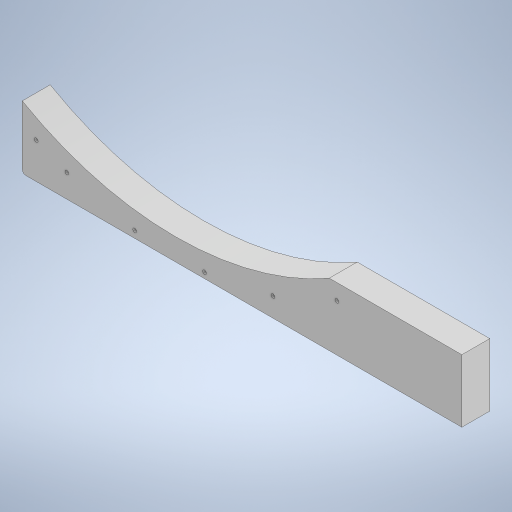
# Autodesk Inventor part: boundaryV1
Saved by Autodesk Inventor 2024.4 (Build 284460000, 460)
## iProperties
Created: 2025-11-05
Part Number: boundaryV1
Material: Generic
Document SubType Name: Modeling
Designer: jonas
Density: 1 g/cm^3
Appearance: Default
Author: jonas
Autodesk Inventor part; units mm, degrees
ref_plane "YZ Plane" through (0, 0, 0) normal (1, 0, 0) x (0, 1, 0)
ref_plane "XZ Plane" through (0, 0, 0) normal (0, 1, 0) x (-1, 0, 0)
ref_plane "XY Plane" through (0, 0, 0) normal (0, 0, 1) x (1, 0, 0)
sketch "Sketch1" plane through (0, 0, 0) normal (0, 1, 0) x (-1, 0, 0)
  line L0 (0, 329.241) -> (0, -329.241) construction
  line L1 (203.5937, 0) -> (-203.5937, 0) construction
  arc A0 (-441.1, 0) -> (220, -382.3208) centre (0, 0) ccw
  line L2 (-441.1, 0) -> (-441.1, 400)
  line L3 (-441.1, 400) -> (-500, 400)
  line L4 (-500, 400) -> (-500, -500)
  line L5 (-500, -500) -> (220, -500)
  line L6 (220, -500) -> (220, -382.3208)
  dimension "d0" = 500
  dimension "d1" = 400
  dimension "d2" = 500
  dimension "d3" = 441.1
  dimension "d4" = 720
  constraints: 14 end point, 3 perpendicular, 2 coincident, 2 midpoint, 2 point on circle, 2 vertical, 1 centre point, 1 horizontal, 1 tangent
  measures "d0" distance between parallel lines of L4 L0
  measures "d1" distance between parallel lines of L3 L1
  measures "d2" distance between parallel lines of L5 L1
  measures "d3" radius of A0
  measures "d4" distance between parallel lines of L4 L6
extrude "Extrusion1" add sketch "Sketch1" along normal blind 40
sketch "Sketch3" plane through (0, 0, 0) normal (0, -1, 0) x (1, 0, 0)
  line L0 (-480, -472.3208) -> (410, -472.3208)
  line L1 (410, -472.3208) -> (410, -382.3208)
  line L2 (410, -382.3208) -> (-480, -382.3208)
  line L3 (-480, -382.3208) -> (-480, -472.3208)
  arc A0 (-220, -382.3208) -> (441.1, 0) centre (0, 0) ccw projected
  line L4 (500, 400) -> (500, -500) projected
  line L5 (-944.7434, 629.3425) -> (927.6453, 629.3425)
  line L6 (927.6453, 629.3425) -> (927.6453, -768.0218)
  line L7 (927.6453, -768.0218) -> (-944.7434, -768.0218)
  line L8 (-944.7434, -768.0218) -> (-944.7434, 629.3425)
  dimension "d44" = 890
  dimension "d45" = 90
  dimension "d71" = 90
  constraints: 16 end point, 4 parallel, 2 horizontal, 2 perpendicular, 1 point on line
  measures "d44" distance of L1.end L2.end
  measures "d45" distance of L2.end L0.start
  measures "d71" distance between parallel lines of L4 L1
sketch "Sketch4" plane through (0, 0, 0) normal (0, -1, 0) x (1, 0, 0)
  line L0 (441.1, 400) -> (500, 400) construction
  line L1 (441.1, 0) -> (441.1, 400) construction
  arc A0 (-220, -382.3208) -> (441.1, 0) centre (0, 0) ccw construction
  line L2 (464.3817, -39.9852) -> (0, 0) construction
  line L3 (0, 0) -> (445.1648, -138.1214) construction
  line L4 (423.7332, -194.1633) -> (0, 0) construction
  line L5 (360.2723, -295.7246) -> (0, 0) construction
  line L6 (289.0138, -365.6778) -> (0, 0) construction
  line L7 (389.8771, -255.4312) -> (0, 0) construction
  line L8 (326.5218, -332.615) -> (0, 0) construction
  line L9 (230.9911, -404.8361) -> (0, 0) construction
  line L10 (139.32, -444.7911) -> (0, 0) construction
  line L11 (41.2359, -464.2723) -> (0, 0) construction
  line L12 (464.3817, -39.9852) -> (445.1648, -138.1214) construction
  line L13 (445.1648, -138.1214) -> (423.7332, -194.1633) construction
  line L14 (423.7332, -194.1633) -> (389.8771, -255.4312) construction
  line L15 (389.8771, -255.4312) -> (360.2723, -295.7246) construction
  line L16 (360.2723, -295.7246) -> (326.5218, -332.615) construction
  line L17 (326.5218, -332.615) -> (289.0138, -365.6778) construction
  line L18 (289.0138, -365.6778) -> (230.9911, -404.8361) construction
  line L19 (230.9911, -404.8361) -> (139.32, -444.7911) construction
  line L20 (139.32, -444.7911) -> (41.2359, -464.2723) construction
  line L21 (-58.7462, -462.3831) -> (0, 0) construction
  line L22 (-156.0243, -439.2102) -> (0, 0) construction
  line L23 (-200, -421.0098) -> (0, 0) construction
  line L24 (41.2359, -464.2723) -> (-58.7462, -462.3831) construction
  line L25 (-58.7462, -462.3831) -> (-156.0243, -439.2102) construction
  line L26 (-200, -421.0098) -> (-156.0243, -439.2102) construction
  line L27 (-220, -500) -> (-220, -382.3208) construction
  point P0 (466.1, 360)
  point P1 (466.1, 260)
  point P2 (466.1, 160)
  point P3 (466.1, 60)
  dimension "d50" = 40
  dimension "d51" = 100
  dimension "d52" = 100
  dimension "d53" = 100
  dimension "d54" = 25
  dimension "d55" = 466.1
  dimension "d56" = 100
  dimension "d57" = 100
  dimension "d58" = 60
  dimension "d59" = 70
  dimension "d60" = 50
  dimension "d61" = 70
  dimension "d62" = 100
  dimension "d63" = 20
  constraints: 50 end point, 17 equal length, 3 vertical alignment
  measures "d50" distance from line of point (466.1, 360) L0
  measures "d51" distance of point (466.1, 260) point (466.1, 360)
  measures "d52" distance of point (466.1, 260) point (466.1, 160)
  measures "d53" distance of point (466.1, 160) point (466.1, 60)
  measures "d54" distance from line of L1 point (466.1, 360)
  measures "d55" distance of L2.start L2.end
  measures "d56" distance of L2.start L3.end
  measures "d57" distance of point (466.1, 60) L2.start
  measures "d58" distance of L3.end L4.start
  measures "d59" distance of L4.start L7.start
  measures "d60" distance of L5.start L8.start
  measures "d61" distance of L9.start L6.start
  measures "d62" distance of L9.start L10.start
  measures "d63" distance from line of L27 L23.start
hole "Hole1" at (-200, 0, -421.0098) at (-156.0243, 0, -439.2102) at (-58.7462, 0, -462.3831) at (41.2359, 0, -464.2723) at (139.32, 0, -444.7911) at (230.9911, 0, -404.8361) at (289.0138, 0, -365.6778) at (326.5218, 0, -332.615) at (360.2723, 0, -295.7246) at (389.8771, 0, -255.4312) at (423.7332, 0, -194.1633) at (445.1648, 0, -138.1214) at (464.3817, 0, -39.9852) at (466.1, 0, 60) at (466.1, 0, 160) at (466.1, 0, 260) at (466.1, 0, 360) direction (0, 1, 0) diameter 5.5 end through all clearance for "Countersunk Flat Head Screw DIN EN ISO 2009" size "M5" standard "DIN"
extrude "Extrusion2" cut sketch "Sketch3" against normal through all
fillet "Fillet1" radius 5 1 edges at (-220, 20, -472.3208)
body "Solid1"
